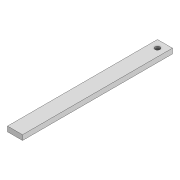
# Autodesk Inventor part: Cable_tie_CF
Saved by Autodesk Inventor 2022 (Build 260153000, 153)
## iProperties
Created: 2022-09-18
Part Number: Cable_tie_CF
Material: Generic
Document SubType Name: Modeling
Designer: dell
Density: 1 g/cm^3
Appearance: Default
Author: dell
Autodesk Inventor part; units mm, degrees
ref_plane "YZ Plane" through (0, 0, 0) normal (1, 0, 0) x (0, 1, 0)
ref_plane "XZ Plane" through (0, 0, 0) normal (0, 1, 0) x (-1, 0, 0)
ref_plane "XY Plane" through (0, 0, 0) normal (0, 0, 1) x (1, 0, 0)
sketch "Sketch1" plane through (0, 0, 0) normal (0, 1, 0) x (-1, 0, 0)
  line L0 (0, 0) -> (6, 0)
  line L1 (6, 0) -> (6, -60)
  line L2 (6, -60) -> (0, -60)
  line L3 (0, -60) -> (0, 0)
  circle A0 centre (3, -57) radius 1
  dimension "d0" = 60
  dimension "d1" = 6
  dimension "d2" = 2
  dimension "d4" = 2
  dimension "d5" = 3
  constraints: 8 end point, 2 parallel, 1 centre point, 1 horizontal, 1 perpendicular
  measures "d0" distance of L2.end L0.start
  measures "d1" distance between parallel lines of L3 L1
  measures "d2" diameter of A0
  measures "d4" distance edge to line of A0 L2
  measures "d5" distance from line of L3 A0.centre
extrude "Extrusion1" add sketch "Sketch1" along normal blind 2
body "Solid1"
